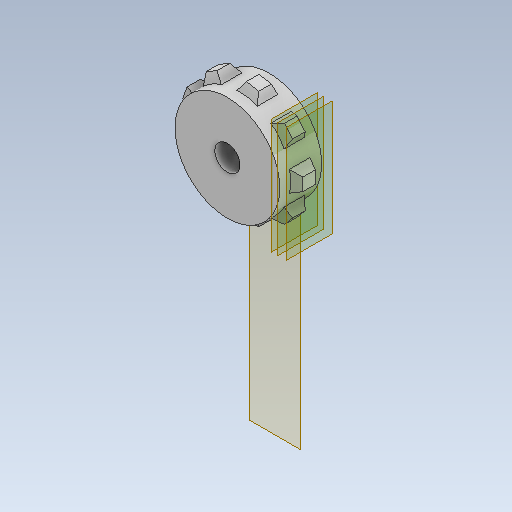
# Autodesk Inventor part: wheel
Saved by Autodesk Inventor 2020 (Build 240168000, 168)
## iProperties
Created: 2020-04-12
Part Number: wheel
Material: Ogólny
Document SubType Name: Modeling
Designer: blep
Density: 1 g/cm^3
Appearance: Domyślna
Author: blep
Autodesk Inventor part; units mm, degrees
ref_plane "YZ Plane" through (0, 0, 0) normal (1, 0, 0) x (0, 1, 0)
ref_plane "XZ Plane" through (0, 0, 0) normal (0, 1, 0) x (-1, 0, 0)
ref_plane "XY Plane" through (0, 0, 0) normal (0, 0, 1) x (1, 0, 0)
ref_plane "Płaszczyzna konstrukcyjna1" through (-6.2, -86.5, 1) normal (0, 0, 1) x (0, -1, 0)
sketch "Szkic1" plane through (-6.2, -86.5, 1) normal (0, 0, 1) x (0, -1, 0)
  arc A0 (-89.8717, 0.5902) -> (-95.3722, 1.2373) centre (-92, 6.2) ccw construction
  circle A1 centre (-92, 6.2) radius 10
  circle A2 centre (-92, 6.2) radius 25
  point P0 (-86.5, 6.2)
  dimension "d0" = 20
  dimension "d1" = 50
  constraints: 2 centre point, 2 coincident
  measures "d0" diameter of A1
  measures "d1" diameter of A2
extrude "Wyciągnięcie proste1" add sketch "Szkic1" along normal blind 20
ref_plane "Płaszczyzna konstrukcyjna2" through (0, 4.593, 6) normal (0, 0, 1) x (1, 0, 0)
sketch "Szkic3" plane through (0, 5.5, 21) normal (0, 0, 1) x (1, 0, 0)
  circle A0 centre (0, 0) radius 10 projected
  point P0 (0, -5.5)
extrude "Wyciągnięcie proste2" add sketch "Szkic3" against normal up to surface (20 mm away)
sketch "Szkic4" plane through (0, 5.5, 21) normal (0, 0, 1) x (1, 0, 0)
  circle A0 centre (0, 0) radius 25 construction
  circle A1 centre (0, 0) radius 2.25
  point P0 (0, -5.5)
  dimension "d6" = 4.5
  constraints: 1 centre point, 1 coincident
  measures "d6" diameter of A1
extrude "Wyciągnięcie proste3" cut sketch "Szkic4" against normal through all
ref_plane "Płaszczyzna konstrukcyjna4" through (25, 5.5, 1) normal (-1, 0, 0) x (0, -1, 0)
ref_plane "Płaszczyzna konstrukcyjna3" through (-8.2, -33.5, -38) normal (-1, 0, 0) x (0, 1, 0)
ref_plane "Płaszczyzna konstrukcyjna5" through (22, 5.5, 1) normal (-1, 0, 0) x (0, -1, 0)
sketch "Szkic5" plane through (22, 5.5, 1) normal (-1, 0, 0) x (0, -1, 0)
  line L0 (25, 0) -> (-25, 0) construction
  line L1 (25, 20) -> (-25, 20) construction
  line L2 (-25, 0) -> (-25, 20) construction
  line L3 (25, 0) -> (25, 20) construction
  line L4 (-6, 4) -> (6, 4)
  line L5 (6, 4) -> (6, 16)
  line L6 (6, 16) -> (-6, 16)
  line L7 (-6, 16) -> (-6, 4)
  line L8 (-6, 4) -> (-6, 0) construction
  line L9 (-6, 16) -> (-6, 20) construction
  line L10 (-6, 16) -> (-25, 16) construction
  line L11 (6, 16) -> (25, 16) construction
  point P0 (5.5, -1)
  dimension "d10" = 12
  dimension "d11" = 12
  constraints: 16 end point, 4 point on line, 3 horizontal, 2 collinear, 2 parallel, 2 vertical, 1 perpendicular
  measures "d10" distance of L4.end L5.end
  measures "d11" distance of L5.end L6.end
ref_plane "Płaszczyzna konstrukcyjna6" through (29, 5.5, 1) normal (-1, 0, 0) x (0, -1, 0)
sketch "Szkic6" plane through (29, 5.5, 1) normal (-1, 0, 0) x (0, -1, 0)
  line L0 (-6, 4) -> (6, 4) construction
  line L1 (6, 16) -> (-6, 16) construction
  line L2 (-6, 16) -> (-6, 4) construction
  line L3 (6, 4) -> (6, 16) construction
  line L4 (3, 7) -> (-3, 7)
  line L5 (-3, 7) -> (-3, 13)
  line L6 (-3, 13) -> (3, 13)
  line L7 (3, 13) -> (3, 7)
  point P0 (5.5, -1)
  dimension "d13" = 3
  constraints: 8 end point, 3 other
  measures "d13" distance between parallel lines of L0 L4
loft "Wyciągnięcie złożone1" add profiles "Szkic5", "Szkic6"
pattern_circular "Szyk kołowy1" count 9 over 360 about axis through (0, 5.5, 21) along (0, 0, -1) of "Wyciągnięcie złożone1"
sketch "Szkic8" plane through (0, 5.5, 1) normal (0, 0, -1) x (-1, 0, 0)
  circle A0 centre (0, 0) radius 2.25 projected
  circle A1 centre (0, 0) radius 25
  circle A2 centre (0, 0) radius 25 projected
  point P0 (0, -5.5)
  constraints: 1 centre point, 1 coincident, 1 concentric
extrude "Wyciągnięcie proste5" add sketch "Szkic8" along normal blind 7.6
spur gear teeth "Przekładnia walcowa2" teeth 24 pitch diameter 27 tip diameter 28.0659 root diameter 23.3008 face width 8 trims to tip circle yes start plane through (0, 5.5, -6.6) normal (0, 0, -1) x (-1, 0, 0)
sketch "Szkic9" plane through (0, 5.5, -6.6) normal (0, 0, -1) x (-1, 0, 0)
  arc A0 (7.4104, 11.9168) -> (6.6151, 12.376) centre (0, 0) ccw projected
  arc A1 (6.6151, 12.376) -> (4.8082, 10.6119) centre (12.3251, 4.7199) ccw projected
  arc A2 (4.8082, 10.6119) -> (4.1038, 10.9037) centre (0, 0) ccw projected
  arc A3 (4.1038, 10.9037) -> (4.0736, 13.4287) centre (-5.3777, 12.0526) ccw projected
  arc A4 (4.0736, 13.4287) -> (3.1866, 13.6664) centre (0, 0) ccw projected
  arc A5 (3.1866, 13.6664) -> (1.8978, 11.4948) centre (10.6836, 7.749) ccw projected
  arc A6 (1.8978, 11.4948) -> (1.1419, 11.5943) centre (0, 0) ccw projected
  arc A7 (1.1419, 11.5943) -> (0.4591, 14.0254) centre (-8.3139, 10.2501) ccw projected
  arc A8 (0.4591, 14.0254) -> (-0.4591, 14.0254) centre (0, 0) ccw projected
  arc A9 (-0.4591, 14.0254) -> (-1.1419, 11.5943) centre (8.3139, 10.2501) ccw projected
  arc A10 (-1.1419, 11.5943) -> (-1.8978, 11.4948) centre (0, 0) ccw projected
  arc A11 (-1.8978, 11.4948) -> (-3.1866, 13.6664) centre (-10.6836, 7.749) ccw projected
  arc A12 (-3.1866, 13.6664) -> (-4.0736, 13.4287) centre (0, 0) ccw projected
  arc A13 (-4.0736, 13.4287) -> (-4.1038, 10.9037) centre (5.3777, 12.0526) ccw projected
  arc A14 (-4.1038, 10.9037) -> (-4.8082, 10.6119) centre (0, 0) ccw projected
  arc A15 (-4.8082, 10.6119) -> (-6.6151, 12.376) centre (-12.3251, 4.7199) ccw projected
  arc A16 (-6.6151, 12.376) -> (-7.4104, 11.9168) centre (0, 0) ccw projected
  arc A17 (-7.4104, 11.9168) -> (-6.7861, 9.47) centre (2.075, 13.0338) ccw projected
  arc A18 (-6.7861, 9.47) -> (-7.3909, 9.0059) centre (0, 0) ccw projected
  arc A19 (-7.3909, 9.0059) -> (-9.5928, 10.2422) centre (-13.1267, 1.3691) ccw projected
  arc A20 (-9.5928, 10.2422) -> (-10.2422, 9.5928) centre (0, 0) ccw projected
  arc A21 (-10.2422, 9.5928) -> (-9.0059, 7.3909) centre (-1.3691, 13.1267) ccw projected
  arc A22 (-9.0059, 7.3909) -> (-9.47, 6.7861) centre (0, 0) ccw projected
  arc A23 (-9.47, 6.7861) -> (-11.9168, 7.4104) centre (-13.0338, -2.075) ccw projected
  arc A24 (-11.9168, 7.4104) -> (-12.376, 6.6151) centre (0, 0) ccw projected
  arc A25 (-12.376, 6.6151) -> (-10.6119, 4.8082) centre (-4.7199, 12.3251) ccw projected
  arc A26 (-10.6119, 4.8082) -> (-10.9037, 4.1038) centre (0, 0) ccw projected
  arc A27 (-10.9037, 4.1038) -> (-13.4287, 4.0736) centre (-12.0526, -5.3777) ccw projected
  arc A28 (-13.4287, 4.0736) -> (-13.6664, 3.1866) centre (0, 0) ccw projected
  arc A29 (-13.6664, 3.1866) -> (-11.4948, 1.8978) centre (-7.749, 10.6836) ccw projected
  arc A30 (-11.4948, 1.8978) -> (-11.5943, 1.1419) centre (0, 0) ccw projected
  arc A31 (-11.5943, 1.1419) -> (-14.0254, 0.4591) centre (-10.2501, -8.3139) ccw projected
  arc A32 (-14.0254, 0.4591) -> (-14.0254, -0.4591) centre (0, 0) ccw projected
  arc A33 (-14.0254, -0.4591) -> (-11.5943, -1.1419) centre (-10.2501, 8.3139) ccw projected
  arc A34 (-11.5943, -1.1419) -> (-11.4948, -1.8978) centre (0, 0) ccw projected
  arc A35 (-11.4948, -1.8978) -> (-13.6664, -3.1866) centre (-7.749, -10.6836) ccw projected
  arc A36 (-13.6664, -3.1866) -> (-13.4287, -4.0736) centre (0, 0) ccw projected
  arc A37 (-13.4287, -4.0736) -> (-10.9037, -4.1038) centre (-12.0526, 5.3777) ccw projected
  arc A38 (-10.9037, -4.1038) -> (-10.6119, -4.8082) centre (0, 0) ccw projected
  arc A39 (-10.6119, -4.8082) -> (-12.376, -6.6151) centre (-4.7199, -12.3251) ccw projected
  arc A40 (-12.376, -6.6151) -> (-11.9168, -7.4104) centre (0, 0) ccw projected
  arc A41 (-11.9168, -7.4104) -> (-9.47, -6.7861) centre (-13.0338, 2.075) ccw projected
  arc A42 (-9.47, -6.7861) -> (-9.0059, -7.3909) centre (0, 0) ccw projected
  arc A43 (-9.0059, -7.3909) -> (-10.2422, -9.5928) centre (-1.3691, -13.1267) ccw projected
  arc A44 (-10.2422, -9.5928) -> (-9.5928, -10.2422) centre (0, 0) ccw projected
  arc A45 (-9.5928, -10.2422) -> (-7.3909, -9.0059) centre (-13.1267, -1.3691) ccw projected
  arc A46 (-7.3909, -9.0059) -> (-6.7861, -9.47) centre (0, 0) ccw projected
  arc A47 (-6.7861, -9.47) -> (-7.4104, -11.9168) centre (2.075, -13.0338) ccw projected
  arc A48 (-7.4104, -11.9168) -> (-6.6151, -12.376) centre (0, 0) ccw projected
  arc A49 (-6.6151, -12.376) -> (-4.8082, -10.6119) centre (-12.3251, -4.7199) ccw projected
  arc A50 (-4.8082, -10.6119) -> (-4.1038, -10.9037) centre (0, 0) ccw projected
  arc A51 (-4.1038, -10.9037) -> (-4.0736, -13.4287) centre (5.3777, -12.0526) ccw projected
  arc A52 (-4.0736, -13.4287) -> (-3.1866, -13.6664) centre (0, 0) ccw projected
  arc A53 (-3.1866, -13.6664) -> (-1.8978, -11.4948) centre (-10.6836, -7.749) ccw projected
  arc A54 (-1.8978, -11.4948) -> (-1.1419, -11.5943) centre (0, 0) ccw projected
  arc A55 (-1.1419, -11.5943) -> (-0.4591, -14.0254) centre (8.3139, -10.2501) ccw projected
  arc A56 (-0.4591, -14.0254) -> (0.4591, -14.0254) centre (0, 0) ccw projected
  arc A57 (0.4591, -14.0254) -> (1.1419, -11.5943) centre (-8.3139, -10.2501) ccw projected
  arc A58 (1.1419, -11.5943) -> (1.8978, -11.4948) centre (0, 0) ccw projected
  arc A59 (1.8978, -11.4948) -> (3.1866, -13.6664) centre (10.6836, -7.749) ccw projected
  arc A60 (3.1866, -13.6664) -> (4.0736, -13.4287) centre (0, 0) ccw projected
  arc A61 (4.0736, -13.4287) -> (4.1038, -10.9037) centre (-5.3777, -12.0526) ccw projected
  arc A62 (4.1038, -10.9037) -> (4.8082, -10.6119) centre (0, 0) ccw projected
  arc A63 (4.8082, -10.6119) -> (6.6151, -12.376) centre (12.3251, -4.7199) ccw projected
  arc A64 (6.6151, -12.376) -> (7.4104, -11.9168) centre (0, 0) ccw projected
  arc A65 (7.4104, -11.9168) -> (6.7861, -9.47) centre (-2.075, -13.0338) ccw projected
  arc A66 (6.7861, -9.47) -> (7.3909, -9.0059) centre (0, 0) ccw projected
  arc A67 (7.3909, -9.0059) -> (9.5928, -10.2422) centre (13.1267, -1.3691) ccw projected
  arc A68 (9.5928, -10.2422) -> (10.2422, -9.5928) centre (0, 0) ccw projected
  arc A69 (10.2422, -9.5928) -> (9.0059, -7.3909) centre (1.3691, -13.1267) ccw projected
  arc A70 (9.0059, -7.3909) -> (9.47, -6.7861) centre (0, 0) ccw projected
  arc A71 (9.47, -6.7861) -> (11.9168, -7.4104) centre (13.0338, 2.075) ccw projected
  arc A72 (11.9168, -7.4104) -> (12.376, -6.6151) centre (0, 0) ccw projected
  arc A73 (12.376, -6.6151) -> (10.6119, -4.8082) centre (4.7199, -12.3251) ccw projected
  arc A74 (10.6119, -4.8082) -> (10.9037, -4.1038) centre (0, 0) ccw projected
  arc A75 (10.9037, -4.1038) -> (13.4287, -4.0736) centre (12.0526, 5.3777) ccw projected
  arc A76 (13.4287, -4.0736) -> (13.6664, -3.1866) centre (0, 0) ccw projected
  arc A77 (13.6664, -3.1866) -> (11.4948, -1.8978) centre (7.749, -10.6836) ccw projected
  arc A78 (11.4948, -1.8978) -> (11.5943, -1.1419) centre (0, 0) ccw projected
  arc A79 (11.5943, -1.1419) -> (14.0254, -0.4591) centre (10.2501, 8.3139) ccw projected
  arc A80 (14.0254, -0.4591) -> (14.0254, 0.4591) centre (0, 0) ccw projected
  arc A81 (14.0254, 0.4591) -> (11.5943, 1.1419) centre (10.2501, -8.3139) ccw projected
  arc A82 (11.5943, 1.1419) -> (11.4948, 1.8978) centre (0, 0) ccw projected
  arc A83 (11.4948, 1.8978) -> (13.6664, 3.1866) centre (7.749, 10.6836) ccw projected
  arc A84 (13.6664, 3.1866) -> (13.4287, 4.0736) centre (0, 0) ccw projected
  arc A85 (13.4287, 4.0736) -> (10.9037, 4.1038) centre (12.0526, -5.3777) ccw projected
  arc A86 (10.9037, 4.1038) -> (10.6119, 4.8082) centre (0, 0) ccw projected
  arc A87 (10.6119, 4.8082) -> (12.376, 6.6151) centre (4.7199, 12.3251) ccw projected
  arc A88 (12.376, 6.6151) -> (11.9168, 7.4104) centre (0, 0) ccw projected
  arc A89 (11.9168, 7.4104) -> (9.47, 6.7861) centre (13.0338, -2.075) ccw projected
  arc A90 (9.47, 6.7861) -> (9.0059, 7.3909) centre (0, 0) ccw projected
  arc A91 (9.0059, 7.3909) -> (10.2422, 9.5928) centre (1.3691, 13.1267) ccw projected
  arc A92 (10.2422, 9.5928) -> (9.5928, 10.2422) centre (0, 0) ccw projected
  arc A93 (9.5928, 10.2422) -> (7.3909, 9.0059) centre (13.1267, 1.3691) ccw projected
  arc A94 (7.3909, 9.0059) -> (6.7861, 9.47) centre (0, 0) ccw projected
  arc A95 (6.7861, 9.47) -> (7.4104, 11.9168) centre (-2.075, 13.0338) ccw projected
  circle A96 centre (0, 0) radius 2.25 projected
  arc A97 (-6.6195, -12.3168) -> (-4.8234, -10.5501) centre (-12.3251, -4.7199) ccw
  arc A98 (-7.3569, -11.8911) -> (-6.6195, -12.3168) centre (0, 0) ccw
  arc A99 (-6.725, -9.4522) -> (-7.3569, -11.8911) centre (2.075, -13.0338) ccw
  arc A100 (-7.3896, -8.9422) -> (-6.725, -9.4522) centre (0, 0) ccw
  arc A101 (-9.5818, -10.1839) -> (-7.3896, -8.9422) centre (-13.1267, -1.3691) ccw
  arc A102 (-10.1839, -9.5818) -> (-9.5818, -10.1839) centre (0, 0) ccw
  arc A103 (-8.9422, -7.3896) -> (-10.1839, -9.5818) centre (-1.3691, -13.1267) ccw
  arc A104 (-9.4522, -6.725) -> (-8.9422, -7.3896) centre (0, 0) ccw
  arc A105 (-11.8911, -7.3569) -> (-9.4522, -6.725) centre (-13.0338, 2.075) ccw
  arc A106 (-12.3168, -6.6195) -> (-11.8911, -7.3569) centre (0, 0) ccw
  arc A107 (-10.5501, -4.8234) -> (-12.3168, -6.6195) centre (-4.7199, -12.3251) ccw
  arc A108 (-10.8707, -4.0494) -> (-10.5501, -4.8234) centre (0, 0) ccw
  arc A109 (-13.3901, -4.0286) -> (-10.8707, -4.0494) centre (-12.0526, 5.3777) ccw
  arc A110 (-13.6104, -3.2062) -> (-13.3901, -4.0286) centre (0, 0) ccw
  arc A111 (-11.439, -1.9284) -> (-13.6104, -3.2062) centre (-7.749, -10.6836) ccw
  arc A112 (-11.5483, -1.0979) -> (-11.439, -1.9284) centre (0, 0) ccw
  arc A113 (-13.9765, -0.4257) -> (-11.5483, -1.0979) centre (-10.2501, 8.3139) ccw
  arc A114 (-13.9765, 0.4257) -> (-13.9765, -0.4257) centre (0, 0) ccw
  arc A115 (-11.5483, 1.0979) -> (-13.9765, 0.4257) centre (-10.2501, -8.3139) ccw
  arc A116 (-11.439, 1.9284) -> (-11.5483, 1.0979) centre (0, 0) ccw
  arc A117 (-13.6104, 3.2062) -> (-11.439, 1.9284) centre (-7.749, 10.6836) ccw
  arc A118 (-13.3901, 4.0286) -> (-13.6104, 3.2062) centre (0, 0) ccw
  arc A119 (-10.8707, 4.0494) -> (-13.3901, 4.0286) centre (-12.0526, -5.3777) ccw
  arc A120 (-10.5501, 4.8234) -> (-10.8707, 4.0494) centre (0, 0) ccw
  arc A121 (-12.3168, 6.6195) -> (-10.5501, 4.8234) centre (-4.7199, 12.3251) ccw
  arc A122 (-11.8911, 7.3569) -> (-12.3168, 6.6195) centre (0, 0) ccw
  arc A123 (-9.4522, 6.725) -> (-11.8911, 7.3569) centre (-13.0338, -2.075) ccw
  arc A124 (-8.9422, 7.3896) -> (-9.4522, 6.725) centre (0, 0) ccw
  arc A125 (-10.1839, 9.5818) -> (-8.9422, 7.3896) centre (-1.3691, 13.1267) ccw
  arc A126 (-9.5818, 10.1839) -> (-10.1839, 9.5818) centre (0, 0) ccw
  arc A127 (-7.3896, 8.9422) -> (-9.5818, 10.1839) centre (-13.1267, 1.3691) ccw
  arc A128 (-6.725, 9.4522) -> (-7.3896, 8.9422) centre (0, 0) ccw
  arc A129 (-7.3569, 11.8911) -> (-6.725, 9.4522) centre (2.075, 13.0338) ccw
  arc A130 (-6.6195, 12.3168) -> (-7.3569, 11.8911) centre (0, 0) ccw
  arc A131 (-4.8234, 10.5501) -> (-6.6195, 12.3168) centre (-12.3251, 4.7199) ccw
  arc A132 (-4.0494, 10.8707) -> (-4.8234, 10.5501) centre (0, 0) ccw
  arc A133 (-4.0286, 13.3901) -> (-4.0494, 10.8707) centre (5.3777, 12.0526) ccw
  arc A134 (-3.2062, 13.6104) -> (-4.0286, 13.3901) centre (0, 0) ccw
  arc A135 (-1.9284, 11.439) -> (-3.2062, 13.6104) centre (-10.6836, 7.749) ccw
  arc A136 (-1.0979, 11.5483) -> (-1.9284, 11.439) centre (0, 0) ccw
  arc A137 (-0.4257, 13.9765) -> (-1.0979, 11.5483) centre (8.3139, 10.2501) ccw
  arc A138 (0.4257, 13.9765) -> (-0.4257, 13.9765) centre (0, 0) ccw
  arc A139 (1.0979, 11.5483) -> (0.4257, 13.9765) centre (-8.3139, 10.2501) ccw
  arc A140 (1.9284, 11.439) -> (1.0979, 11.5483) centre (0, 0) ccw
  arc A141 (3.2062, 13.6104) -> (1.9284, 11.439) centre (10.6836, 7.749) ccw
  arc A142 (4.0286, 13.3901) -> (3.2062, 13.6104) centre (0, 0) ccw
  arc A143 (4.0494, 10.8707) -> (4.0286, 13.3901) centre (-5.3777, 12.0526) ccw
  arc A144 (4.8234, 10.5501) -> (4.0494, 10.8707) centre (0, 0) ccw
  arc A145 (6.6195, 12.3168) -> (4.8234, 10.5501) centre (12.3251, 4.7199) ccw
  arc A146 (7.3569, 11.8911) -> (6.6195, 12.3168) centre (0, 0) ccw
  arc A147 (6.725, 9.4522) -> (7.3569, 11.8911) centre (-2.075, 13.0338) ccw
  arc A148 (7.3896, 8.9422) -> (6.725, 9.4522) centre (0, 0) ccw
  arc A149 (9.5818, 10.1839) -> (7.3896, 8.9422) centre (13.1267, 1.3691) ccw
  arc A150 (10.1839, 9.5818) -> (9.5818, 10.1839) centre (0, 0) ccw
  arc A151 (8.9422, 7.3896) -> (10.1839, 9.5818) centre (1.3691, 13.1267) ccw
  arc A152 (9.4522, 6.725) -> (8.9422, 7.3896) centre (0, 0) ccw
  arc A153 (11.8911, 7.3569) -> (9.4522, 6.725) centre (13.0338, -2.075) ccw
  arc A154 (12.3168, 6.6195) -> (11.8911, 7.3569) centre (0, 0) ccw
  arc A155 (10.5501, 4.8234) -> (12.3168, 6.6195) centre (4.7199, 12.3251) ccw
  arc A156 (10.8707, 4.0494) -> (10.5501, 4.8234) centre (0, 0) ccw
  arc A157 (13.3901, 4.0286) -> (10.8707, 4.0494) centre (12.0526, -5.3777) ccw
  arc A158 (13.6104, 3.2062) -> (13.3901, 4.0286) centre (0, 0) ccw
  arc A159 (11.439, 1.9284) -> (13.6104, 3.2062) centre (7.749, 10.6836) ccw
  arc A160 (11.5483, 1.0979) -> (11.439, 1.9284) centre (0, 0) ccw
  arc A161 (13.9765, 0.4257) -> (11.5483, 1.0979) centre (10.2501, -8.3139) ccw
  arc A162 (13.9765, -0.4257) -> (13.9765, 0.4257) centre (0, 0) ccw
  arc A163 (11.5483, -1.0979) -> (13.9765, -0.4257) centre (10.2501, 8.3139) ccw
  arc A164 (11.439, -1.9284) -> (11.5483, -1.0979) centre (0, 0) ccw
  arc A165 (13.6104, -3.2062) -> (11.439, -1.9284) centre (7.749, -10.6836) ccw
  arc A166 (13.3901, -4.0286) -> (13.6104, -3.2062) centre (0, 0) ccw
  arc A167 (10.8707, -4.0494) -> (13.3901, -4.0286) centre (12.0526, 5.3777) ccw
  arc A168 (10.5501, -4.8234) -> (10.8707, -4.0494) centre (0, 0) ccw
  arc A169 (12.3168, -6.6195) -> (10.5501, -4.8234) centre (4.7199, -12.3251) ccw
  arc A170 (11.8911, -7.3569) -> (12.3168, -6.6195) centre (0, 0) ccw
  arc A171 (9.4522, -6.725) -> (11.8911, -7.3569) centre (13.0338, 2.075) ccw
  arc A172 (8.9422, -7.3896) -> (9.4522, -6.725) centre (0, 0) ccw
  arc A173 (10.1839, -9.5818) -> (8.9422, -7.3896) centre (1.3691, -13.1267) ccw
  arc A174 (9.5818, -10.1839) -> (10.1839, -9.5818) centre (0, 0) ccw
  arc A175 (7.3896, -8.9422) -> (9.5818, -10.1839) centre (13.1267, -1.3691) ccw
  arc A176 (6.725, -9.4522) -> (7.3896, -8.9422) centre (0, 0) ccw
  arc A177 (7.3569, -11.8911) -> (6.725, -9.4522) centre (-2.075, -13.0338) ccw
  arc A178 (6.6195, -12.3168) -> (7.3569, -11.8911) centre (0, 0) ccw
  arc A179 (4.8234, -10.5501) -> (6.6195, -12.3168) centre (12.3251, -4.7199) ccw
  arc A180 (4.0494, -10.8707) -> (4.8234, -10.5501) centre (0, 0) ccw
  arc A181 (4.0286, -13.3901) -> (4.0494, -10.8707) centre (-5.3777, -12.0526) ccw
  arc A182 (3.2062, -13.6104) -> (4.0286, -13.3901) centre (0, 0) ccw
  arc A183 (1.9284, -11.439) -> (3.2062, -13.6104) centre (10.6836, -7.749) ccw
  arc A184 (1.0979, -11.5483) -> (1.9284, -11.439) centre (0, 0) ccw
  arc A185 (0.4257, -13.9765) -> (1.0979, -11.5483) centre (-8.3139, -10.2501) ccw
  arc A186 (-0.4257, -13.9765) -> (0.4257, -13.9765) centre (0, 0) ccw
  arc A187 (-1.0979, -11.5483) -> (-0.4257, -13.9765) centre (8.3139, -10.2501) ccw
  arc A188 (-1.9284, -11.439) -> (-1.0979, -11.5483) centre (0, 0) ccw
  arc A189 (-3.2062, -13.6104) -> (-1.9284, -11.439) centre (-10.6836, -7.749) ccw
  arc A190 (-4.0286, -13.3901) -> (-3.2062, -13.6104) centre (0, 0) ccw
  arc A191 (-4.0494, -10.8707) -> (-4.0286, -13.3901) centre (5.3777, -12.0526) ccw
  arc A192 (-4.8234, -10.5501) -> (-4.0494, -10.8707) centre (0, 0) ccw
  point P0 (0, -5.5)
  dimension "d30" = 0.05
  constraints: 192 point on circle, 96 centre point, 95 other
  measures "d30" radial gap between concentric circles of A49 A97
extrude "Wyciągnięcie proste6" cut sketch "Szkic9" against normal blind 8 contours A95 A94 A93 A92 A91 A90 A89 A88 A87 A86 A85 A84 A83 A82 A81 A80 A79 A78 A77 A76 A75 A74 A73 A72 A71 A70 A69 A68 A67 A66 A65 A64 A63 A62 A61 A60 A59 A58 A57 A56 A55 A54 A53 A52 A51 A50 A49 A48 A47 A46 A45 A44 A43 A42 A41 A40 A39 A38 A37 A36 A35 A34 A33 A32 A31 A30 A29 A28 A27 A26 A25 A24 A23 A22 A21 A20 A19 A18 A17 A16 A15 A14 A13 A12 A11 A10 A9 A8 A7 A6 A5 A4 A3 A2 A1 A0
sketch "Szkic10" plane through (0, 5.5, 21) normal (0, 0, 1) x (1, 0, 0)
  circle A0 centre (0, 0) radius 2.25 projected
  circle A1 centre (0, 0) radius 6
  point P0 (0, -5.5)
  dimension "d33" = 12
  constraints: 1 centre point, 1 coincident
  measures "d33" diameter of A1
sketch "Szkic11" plane through (0, 5.5, -6.6) normal (0, 0, -1) x (-1, 0, 0)
  circle A0 centre (0, 0) radius 25 construction
  circle A1 centre (0, 0) radius 10
  point P0 (0, -5.5)
  dimension "d36" = 20
  constraints: 1 centre point, 1 coincident
  measures "d36" diameter of A1
sketch "Szkic12" plane through (0, 5.5, 1.4) normal (0, 0, -1) x (-1, 0, 0)
  arc A0 (-10.8707, -4.0494) -> (-10.5501, -4.8234) centre (0, 0) ccw projected
  arc A1 (-13.3901, -4.0286) -> (-10.8707, -4.0494) centre (-12.0526, 5.3777) ccw projected
  arc A2 (-13.6104, -3.2062) -> (-13.3901, -4.0286) centre (0, 0) ccw projected
  arc A3 (-11.439, -1.9284) -> (-13.6104, -3.2062) centre (-7.749, -10.6836) ccw projected
  arc A4 (-11.5483, -1.0979) -> (-11.439, -1.9284) centre (0, 0) ccw projected
  arc A5 (-13.9765, -0.4257) -> (-11.5483, -1.0979) centre (-10.2501, 8.3139) ccw projected
  arc A6 (-13.9765, 0.4257) -> (-13.9765, -0.4257) centre (0, 0) ccw projected
  arc A7 (-11.5483, 1.0979) -> (-13.9765, 0.4257) centre (-10.2501, -8.3139) ccw projected
  arc A8 (-11.439, 1.9284) -> (-11.5483, 1.0979) centre (0, 0) ccw projected
  arc A9 (-13.6104, 3.2062) -> (-11.439, 1.9284) centre (-7.749, 10.6836) ccw projected
  arc A10 (-13.3901, 4.0286) -> (-13.6104, 3.2062) centre (0, 0) ccw projected
  arc A11 (-10.8707, 4.0494) -> (-13.3901, 4.0286) centre (-12.0526, -5.3777) ccw projected
  arc A12 (-10.5501, 4.8234) -> (-10.8707, 4.0494) centre (0, 0) ccw projected
  arc A13 (-12.3168, 6.6195) -> (-10.5501, 4.8234) centre (-4.7199, 12.3251) ccw projected
  arc A14 (-11.8911, 7.3569) -> (-12.3168, 6.6195) centre (0, 0) ccw projected
  arc A15 (-9.4522, 6.725) -> (-11.8911, 7.3569) centre (-13.0338, -2.075) ccw projected
  arc A16 (-8.9422, 7.3896) -> (-9.4522, 6.725) centre (0, 0) ccw projected
  arc A17 (-10.1839, 9.5818) -> (-8.9422, 7.3896) centre (-1.3691, 13.1267) ccw projected
  arc A18 (-9.5818, 10.1839) -> (-10.1839, 9.5818) centre (0, 0) ccw projected
  arc A19 (-7.3896, 8.9422) -> (-9.5818, 10.1839) centre (-13.1267, 1.3691) ccw projected
  arc A20 (-6.725, 9.4522) -> (-7.3896, 8.9422) centre (0, 0) ccw projected
  arc A21 (-7.3569, 11.8911) -> (-6.725, 9.4522) centre (2.075, 13.0338) ccw projected
  arc A22 (-6.6195, 12.3168) -> (-7.3569, 11.8911) centre (0, 0) ccw projected
  arc A23 (-4.8234, 10.5501) -> (-6.6195, 12.3168) centre (-12.3251, 4.7199) ccw projected
  arc A24 (-4.0494, 10.8707) -> (-4.8234, 10.5501) centre (0, 0) ccw projected
  arc A25 (-4.0286, 13.3901) -> (-4.0494, 10.8707) centre (5.3777, 12.0526) ccw projected
  arc A26 (-3.2062, 13.6104) -> (-4.0286, 13.3901) centre (0, 0) ccw projected
  arc A27 (-1.9284, 11.439) -> (-3.2062, 13.6104) centre (-10.6836, 7.749) ccw projected
  arc A28 (-1.0979, 11.5483) -> (-1.9284, 11.439) centre (0, 0) ccw projected
  arc A29 (-0.4257, 13.9765) -> (-1.0979, 11.5483) centre (8.3139, 10.2501) ccw projected
  arc A30 (0.4257, 13.9765) -> (-0.4257, 13.9765) centre (0, 0) ccw projected
  arc A31 (1.0979, 11.5483) -> (0.4257, 13.9765) centre (-8.3139, 10.2501) ccw projected
  arc A32 (1.9284, 11.439) -> (1.0979, 11.5483) centre (0, 0) ccw projected
  arc A33 (3.2062, 13.6104) -> (1.9284, 11.439) centre (10.6836, 7.749) ccw projected
  arc A34 (4.0286, 13.3901) -> (3.2062, 13.6104) centre (0, 0) ccw projected
  arc A35 (4.0494, 10.8707) -> (4.0286, 13.3901) centre (-5.3777, 12.0526) ccw projected
  arc A36 (4.8234, 10.5501) -> (4.0494, 10.8707) centre (0, 0) ccw projected
  arc A37 (6.6195, 12.3168) -> (4.8234, 10.5501) centre (12.3251, 4.7199) ccw projected
  arc A38 (7.3569, 11.8911) -> (6.6195, 12.3168) centre (0, 0) ccw projected
  arc A39 (6.725, 9.4522) -> (7.3569, 11.8911) centre (-2.075, 13.0338) ccw projected
  arc A40 (7.3896, 8.9422) -> (6.725, 9.4522) centre (0, 0) ccw projected
  arc A41 (9.5818, 10.1839) -> (7.3896, 8.9422) centre (13.1267, 1.3691) ccw projected
  arc A42 (10.1839, 9.5818) -> (9.5818, 10.1839) centre (0, 0) ccw projected
  arc A43 (8.9422, 7.3896) -> (10.1839, 9.5818) centre (1.3691, 13.1267) ccw projected
  arc A44 (9.4522, 6.725) -> (8.9422, 7.3896) centre (0, 0) ccw projected
  arc A45 (11.8911, 7.3569) -> (9.4522, 6.725) centre (13.0338, -2.075) ccw projected
  arc A46 (12.3168, 6.6195) -> (11.8911, 7.3569) centre (0, 0) ccw projected
  arc A47 (10.5501, 4.8234) -> (12.3168, 6.6195) centre (4.7199, 12.3251) ccw projected
  arc A48 (10.8707, 4.0494) -> (10.5501, 4.8234) centre (0, 0) ccw projected
  arc A49 (13.3901, 4.0286) -> (10.8707, 4.0494) centre (12.0526, -5.3777) ccw projected
  arc A50 (13.6104, 3.2062) -> (13.3901, 4.0286) centre (0, 0) ccw projected
  arc A51 (11.439, 1.9284) -> (13.6104, 3.2062) centre (7.749, 10.6836) ccw projected
  arc A52 (11.5483, 1.0979) -> (11.439, 1.9284) centre (0, 0) ccw projected
  arc A53 (13.9765, 0.4257) -> (11.5483, 1.0979) centre (10.2501, -8.3139) ccw projected
  arc A54 (13.9765, -0.4257) -> (13.9765, 0.4257) centre (0, 0) ccw projected
  arc A55 (11.5483, -1.0979) -> (13.9765, -0.4257) centre (10.2501, 8.3139) ccw projected
  arc A56 (11.439, -1.9284) -> (11.5483, -1.0979) centre (0, 0) ccw projected
  arc A57 (13.6104, -3.2062) -> (11.439, -1.9284) centre (7.749, -10.6836) ccw projected
  arc A58 (13.3901, -4.0286) -> (13.6104, -3.2062) centre (0, 0) ccw projected
  arc A59 (10.8707, -4.0494) -> (13.3901, -4.0286) centre (12.0526, 5.3777) ccw projected
  arc A60 (10.5501, -4.8234) -> (10.8707, -4.0494) centre (0, 0) ccw projected
  arc A61 (12.3168, -6.6195) -> (10.5501, -4.8234) centre (4.7199, -12.3251) ccw projected
  arc A62 (11.8911, -7.3569) -> (12.3168, -6.6195) centre (0, 0) ccw projected
  arc A63 (9.4522, -6.725) -> (11.8911, -7.3569) centre (13.0338, 2.075) ccw projected
  arc A64 (8.9422, -7.3896) -> (9.4522, -6.725) centre (0, 0) ccw projected
  arc A65 (10.1839, -9.5818) -> (8.9422, -7.3896) centre (1.3691, -13.1267) ccw projected
  arc A66 (9.5818, -10.1839) -> (10.1839, -9.5818) centre (0, 0) ccw projected
  arc A67 (7.3896, -8.9422) -> (9.5818, -10.1839) centre (13.1267, -1.3691) ccw projected
  arc A68 (6.725, -9.4522) -> (7.3896, -8.9422) centre (0, 0) ccw projected
  arc A69 (7.3569, -11.8911) -> (6.725, -9.4522) centre (-2.075, -13.0338) ccw projected
  arc A70 (6.6195, -12.3168) -> (7.3569, -11.8911) centre (0, 0) ccw projected
  arc A71 (4.8234, -10.5501) -> (6.6195, -12.3168) centre (12.3251, -4.7199) ccw projected
  arc A72 (4.0494, -10.8707) -> (4.8234, -10.5501) centre (0, 0) ccw projected
  arc A73 (4.0286, -13.3901) -> (4.0494, -10.8707) centre (-5.3777, -12.0526) ccw projected
  arc A74 (3.2062, -13.6104) -> (4.0286, -13.3901) centre (0, 0) ccw projected
  arc A75 (1.9284, -11.439) -> (3.2062, -13.6104) centre (10.6836, -7.749) ccw projected
  arc A76 (1.0979, -11.5483) -> (1.9284, -11.439) centre (0, 0) ccw projected
  arc A77 (0.4257, -13.9765) -> (1.0979, -11.5483) centre (-8.3139, -10.2501) ccw projected
  arc A78 (-0.4257, -13.9765) -> (0.4257, -13.9765) centre (0, 0) ccw projected
  arc A79 (-1.0979, -11.5483) -> (-0.4257, -13.9765) centre (8.3139, -10.2501) ccw projected
  arc A80 (-1.9284, -11.439) -> (-1.0979, -11.5483) centre (0, 0) ccw projected
  arc A81 (-3.2062, -13.6104) -> (-1.9284, -11.439) centre (-10.6836, -7.749) ccw projected
  arc A82 (-4.0286, -13.3901) -> (-3.2062, -13.6104) centre (0, 0) ccw projected
  arc A83 (-4.0494, -10.8707) -> (-4.0286, -13.3901) centre (5.3777, -12.0526) ccw projected
  arc A84 (-4.8234, -10.5501) -> (-4.0494, -10.8707) centre (0, 0) ccw projected
  arc A85 (-6.6195, -12.3168) -> (-4.8234, -10.5501) centre (-12.3251, -4.7199) ccw projected
  arc A86 (-7.3569, -11.8911) -> (-6.6195, -12.3168) centre (0, 0) ccw projected
  arc A87 (-6.725, -9.4522) -> (-7.3569, -11.8911) centre (2.075, -13.0338) ccw projected
  arc A88 (-7.3896, -8.9422) -> (-6.725, -9.4522) centre (0, 0) ccw projected
  arc A89 (-9.5818, -10.1839) -> (-7.3896, -8.9422) centre (-13.1267, -1.3691) ccw projected
  arc A90 (-10.1839, -9.5818) -> (-9.5818, -10.1839) centre (0, 0) ccw projected
  arc A91 (-8.9422, -7.3896) -> (-10.1839, -9.5818) centre (-1.3691, -13.1267) ccw projected
  arc A92 (-9.4522, -6.725) -> (-8.9422, -7.3896) centre (0, 0) ccw projected
  arc A93 (-11.8911, -7.3569) -> (-9.4522, -6.725) centre (-13.0338, 2.075) ccw projected
  arc A94 (-12.3168, -6.6195) -> (-11.8911, -7.3569) centre (0, 0) ccw projected
  arc A95 (-10.5501, -4.8234) -> (-12.3168, -6.6195) centre (-4.7199, -12.3251) ccw projected
  circle A96 centre (0, 0) radius 25 projected
  point P0 (0, -5.5)
extrude "Wyciągnięcie proste8" add sketch "Szkic12" along normal blind 0.4
extrude "Wyciągnięcie proste9" cut sketch "Szkic11" against normal blind 10
extrude "Wyciągnięcie proste10" cut sketch "Szkic10" against normal blind 12.6 contours A0 | A1
